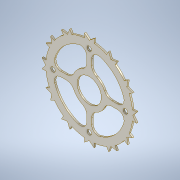
# Autodesk Inventor part: Wood Magnets  (UNI) V1.0.
Saved by Autodesk Inventor 2022.1 (Build 261234020, 234B)
## iProperties
Created: 2022-03-16
Part Number: Wood Magnets  (UNI) V1.0.
Material: Titanium
Document SubType Name: Modeling
Designer: NCai2
Density: 4.51 g/cm^3
Appearance: Titanium
Mass: 5.57938 g
Surface Area: 30.6065 cm^2
Volume: 1.23711 cm^3
Author: NCai2
Autodesk Inventor part; units mm, degrees
ref_plane "YZ Plane" through (0, 0, 0) normal (1, 0, 0) x (0, 1, 0)
ref_plane "XZ Plane" through (0, 0, 0) normal (0, 1, 0) x (-1, 0, 0)
ref_plane "XY Plane" through (0, 0, 0) normal (0, 0, 1) x (1, 0, 0)
sketch "Sketch1" plane through (0, 0, 0) normal (0, 0, 1) x (1, 0, 0)
  circle A0 centre (0, 0) radius 28.575
  circle A1 centre (0, 0) radius 23.8125 construction
  circle A2 centre (0, 0) radius 11.1125
  line L0 (0, 0) -> (0, 28.575) construction
  circle A3 centre (0, 23.8125) radius 1.5
  line L1 (-1.5875, 10.9985) -> (-1.5875, 28.5309)
  line L2 (1.5875, 10.9985) -> (1.5875, 28.5309)
  arc A4 (7.1011, 22.729) -> (1.5875, 18.6752) centre (5.8346, 18.6752) ccw
  arc A5 (-1.5875, 18.6752) -> (-7.1011, 22.729) centre (-5.8346, 18.6752) ccw
  arc A6 (1.5875, 14.919) -> (4.6766, 10.0805) centre (6.9212, 14.919) ccw
  arc A7 (-4.6766, 10.0805) -> (-1.5875, 14.919) centre (-6.9212, 14.919) ccw
  arc A8 (-14.919, 1.5875) -> (-10.0805, 4.6766) centre (-14.919, 6.9212) ccw
  line L3 (-10.9985, 1.5875) -> (-28.5309, 1.5875)
  line L4 (-10.9985, -1.5875) -> (-28.5309, -1.5875)
  arc A9 (-10.0805, -4.6766) -> (-14.919, -1.5875) centre (-14.919, -6.9212) ccw
  arc A10 (-22.729, 7.1011) -> (-18.6752, 1.5875) centre (-18.6752, 5.8346) ccw
  arc A11 (-18.6752, -1.5875) -> (-22.729, -7.1011) centre (-18.6752, -5.8346) ccw
  circle A12 centre (-23.8125, 0) radius 1.5
  arc A13 (-1.5875, -14.919) -> (-4.6766, -10.0805) centre (-6.9212, -14.919) ccw
  line L5 (-1.5875, -10.9985) -> (-1.5875, -28.5309)
  line L6 (1.5875, -10.9985) -> (1.5875, -28.5309)
  arc A14 (4.6766, -10.0805) -> (1.5875, -14.919) centre (6.9212, -14.919) ccw
  arc A15 (-7.1011, -22.729) -> (-1.5875, -18.6752) centre (-5.8346, -18.6752) ccw
  arc A16 (1.5875, -18.6752) -> (7.1011, -22.729) centre (5.8346, -18.6752) ccw
  circle A17 centre (0, -23.8125) radius 1.5
  arc A18 (14.919, -1.5875) -> (10.0805, -4.6766) centre (14.919, -6.9212) ccw
  line L7 (10.9985, -1.5875) -> (28.5309, -1.5875)
  line L8 (10.9985, 1.5875) -> (28.5309, 1.5875)
  arc A19 (10.0805, 4.6766) -> (14.919, 1.5875) centre (14.919, 6.9212) ccw
  arc A20 (22.729, -7.1011) -> (18.6752, -1.5875) centre (18.6752, -5.8346) ccw
  arc A21 (18.6752, 1.5875) -> (22.729, 7.1011) centre (18.6752, 5.8346) ccw
  circle A22 centre (23.8125, 0) radius 1.5
  circle A23 centre (0, 0) radius 7.9375
  arc A24 (-7.1011, 22.729) -> (-22.729, 7.1011) centre (0, 0) ccw
  arc A25 (-23.2345, 5.2148) -> (-17.5143, -16.1334) centre (0, 0) ccw
  arc A26 (-16.1334, -17.5143) -> (5.2148, -23.2345) centre (0, 0) ccw
  arc A27 (7.1011, -22.729) -> (22.729, -7.1011) centre (0, 0) ccw
  arc A28 (23.2345, -5.2148) -> (17.5143, 16.1334) centre (0, 0) ccw
  arc A29 (16.1334, 17.5143) -> (-5.2148, 23.2345) centre (0, 0) ccw
  line L9 (-1.5875, 28.5309) -> (-1.5875, 31.0709) construction
  line L10 (-1.5875, 31.0709) -> (1.5875, 28.5309) construction
  arc A30 (-22.729, -7.1011) -> (-7.1011, -22.729) centre (0, 0) ccw
  arc A31 (7.1011, -22.729) -> (22.729, -7.1011) centre (0, 0) ccw
  arc A32 (23.0011, 6.1631) -> (7.1011, 22.729) centre (0, 0) ccw
  arc A33 (-7.1011, 22.729) -> (-22.729, 7.1011) centre (0, 0) ccw
  line L11 (0, 28.575) -> (-3.175, 28.575) construction
  line L12 (-3.175, 28.575) -> (-3.175, 31.0709) construction
  line L13 (-3.175, 31.0709) -> (0, 31.0709) construction
  line L14 (0, 31.0709) -> (0, 28.575) construction
  line L15 (0, 28.575) -> (-3.175, 31.0709)
  line L16 (-3.175, 28.3981) -> (-3.175, 31.0709)
  line L17 (0, 28.575) -> (3.175, 31.0709)
  line L18 (3.175, 28.3981) -> (3.175, 31.0709)
  line L19 (-14.2875, 24.7467) -> (-12.7858, 28.4957)
  line L20 (-11.4494, 26.1809) -> (-12.7858, 28.4957)
  line L21 (-14.2875, 24.7467) -> (-18.2851, 25.3207)
  line L22 (-16.9487, 23.0059) -> (-18.2851, 25.3207)
  line L23 (-24.7467, 14.2875) -> (-25.3207, 18.2851)
  line L24 (-23.0059, 16.9487) -> (-25.3207, 18.2851)
  line L25 (-24.7467, 14.2875) -> (-28.4957, 12.7858)
  line L26 (-26.1809, 11.4494) -> (-28.4957, 12.7858)
  line L27 (-28.575, 0) -> (-31.0709, 3.175)
  line L28 (-28.3981, 3.175) -> (-31.0709, 3.175)
  line L29 (-28.575, 0) -> (-31.0709, -3.175)
  line L30 (-28.3981, -3.175) -> (-31.0709, -3.175)
  line L31 (-24.7467, -14.2875) -> (-28.4957, -12.7858)
  line L32 (-26.1809, -11.4494) -> (-28.4957, -12.7858)
  line L33 (-24.7467, -14.2875) -> (-25.3207, -18.2851)
  line L34 (-23.0059, -16.9487) -> (-25.3207, -18.2851)
  line L35 (-14.2875, -24.7467) -> (-18.2851, -25.3207)
  line L36 (-16.9487, -23.0059) -> (-18.2851, -25.3207)
  line L37 (-14.2875, -24.7467) -> (-12.7858, -28.4957)
  line L38 (-11.4494, -26.1809) -> (-12.7858, -28.4957)
  line L39 (0, -28.575) -> (-3.175, -31.0709)
  line L40 (-3.175, -28.3981) -> (-3.175, -31.0709)
  line L41 (0, -28.575) -> (3.175, -31.0709)
  line L42 (3.175, -28.3981) -> (3.175, -31.0709)
  line L43 (14.2875, -24.7467) -> (12.7858, -28.4957)
  line L44 (11.4494, -26.1809) -> (12.7858, -28.4957)
  line L45 (14.2875, -24.7467) -> (18.2851, -25.3207)
  line L46 (16.9487, -23.0059) -> (18.2851, -25.3207)
  line L47 (24.7467, -14.2875) -> (25.3207, -18.2851)
  line L48 (23.0059, -16.9487) -> (25.3207, -18.2851)
  line L49 (24.7467, -14.2875) -> (28.4957, -12.7858)
  line L50 (26.1809, -11.4494) -> (28.4957, -12.7858)
  line L51 (28.575, 0) -> (31.0709, -3.175)
  line L52 (28.3981, -3.175) -> (31.0709, -3.175)
  line L53 (28.575, 0) -> (31.0709, 3.175)
  line L54 (28.3981, 3.175) -> (31.0709, 3.175)
  line L55 (24.7467, 14.2875) -> (28.4957, 12.7858)
  line L56 (26.1809, 11.4494) -> (28.4957, 12.7858)
  line L57 (24.7467, 14.2875) -> (25.3207, 18.2851)
  line L58 (23.0059, 16.9487) -> (25.3207, 18.2851)
  line L59 (14.2875, 24.7467) -> (18.2851, 25.3207)
  line L60 (16.9487, 23.0059) -> (18.2851, 25.3207)
  line L61 (14.2875, 24.7467) -> (12.7858, 28.4957)
  line L62 (11.4494, 26.1809) -> (12.7858, 28.4957)
  point P0 (-1.5875, 14.919)
  point P1 (-4.6766, 10.0805)
  point P2 (-10.0805, 4.6766)
  point P3 (-1.5875, 18.6752)
  point P4 (1.5875, -14.919)
  point P5 (4.6766, -10.0805)
  point P6 (10.0805, -4.6766)
  point P7 (-7.072, -22.7381)
  point P8 (-16.1558, -17.4936)
  point P9 (1.5875, -18.6752)
  point P10 (14.919, 1.5875)
  point P11 (10.0805, 4.6766)
  point P12 (7.072, -22.7381)
  point P13 (18.6752, 1.5875)
  point P14 (-14.919, -1.5875)
  point P15 (-10.0805, -4.6766)
  point P16 (-4.6766, -10.0805)
  point P17 (-23.2278, -5.2445)
  point P18 (-22.729, -7.1011)
  point P19 (-18.6752, -1.5875)
  point P20 (7.1011, 22.729)
  point P21 (-23.7595, -1.5875)
  point P22 (16.1334, 17.5143)
  point P23 (17.5143, 16.1334)
  point P24 (22.729, 7.1011)
  point P25 (-7.1011, -22.729)
  point P26 (-16.1334, -17.5143)
  point P27 (-17.5143, -16.1334)
  point P28 (22.729, -7.1011)
  point P29 (7.1011, -22.729)
  point P30 (28.575, 0)
  point P31 (28.575, 0)
  dimension "d0" = 57.15
  dimension "d1" = 47.625
  dimension "d2" = 22.225
  dimension "d3" = 3
  dimension "d4" = 1.5875
  dimension "d5" = 1.5875
  dimension "d8" = 360
  dimension "d10" = 15.875
  dimension "d13" = 360
  dimension "d15" = 2.54
  dimension "d22" = 3.175
  dimension "d25" = 360
  constraints: 126 end point, 60 point on circle, 33 centre point, 10 point on line, 8 symmetric about line, 6 tangent, 5 concentric, 4 coincident, 4 parallel, 2 perpendicular, 2 vertical, 1 horizontal, 1 midpoint, 239 other
  measures "d1" diameter of A1
  measures "d2" diameter of A2
  measures "d3" diameter of A3
  measures "d4" distance between parallel lines of L0 L1
  measures "d5" distance between parallel lines of L0 L2
  measures "d10" diameter of A23
  measures "d15" distance of L1.end L9.end
  measures "d22" distance of L12.end L13.end
extrude "Extrusion1" add sketch "Sketch1" along normal blind 1 contours A0 L7 A28 A22 L8 | L51 L52 A0 | A0 L54 L53 | L8 A28 A32 A29 L2 A0 | A0 L6 A16 A27 A20 L7 | A28 A22 L7 A2 L8 | L8 A21 A28 | A0 L55 L56 | L50 L49 A0 | A0 L58 L57 | L8 A2 A19 | L47 L48 A0 | A18 A2 L7 | A2 | A0 L59 L60 | A2 L2 A6 | L46 L45 A0 | A14 L6 A2 | L6 A26 A17 L5 A2 | A0 L62 L61 | A2 L1 A29 A3 L2 | A4 L2 A29 | L43 L44 A0 | L6 A0 L5 A26 A17 | A2 A7 L1 | A29 A3 L1 A0 L2 | L5 A13 A2 | A0 L42 L41 | A0 L17 L18 | L39 L40 A0 | A2 L3 A8 | A5 A24 A10 L3 A0 L1 | A0 L16 L15 | A9 L4 A2 | L5 A26 A15 | A0 L4 A25 A30 A26 L5 | A2 L4 A25 A12 L3 | A11 A25 L4 | L38 L37 A0 | A25 A12 L4 A0 L3 | A0 L19 L20 | L35 L36 A0 | A0 L27 L28 | A0 L22 L21 | A0 L30 L29 | L34 L33 A0 | L26 L25 A0 | A0 L23 L24 | A0 L31 L32
body "Solid1"
